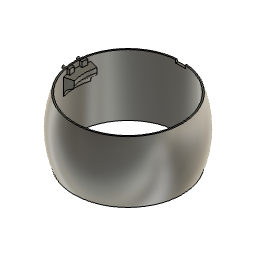
sphere_PS4_USB_C v6 (Autodesk Fusion 360 design; units mm, degrees)
Autodesk Fusion 360 part; units mm, degrees
note: some values were not read from the file. Set by a fixed rule: which face or edge a step refers to.
ref_plane "Arbeitsebene2" through (0, 0, 70) normal (0, 0, 1) x (1, 0, 0)
sketch "Skizze1" plane through (0, 0, 70) normal (0, 0, 1) x (1, 0, 0)
  circle A0 centre (0, 0) radius 60
  line L0 (-32, -65.4497) -> (-32, 74.1763) construction
  line L1 (32, -65.9786) -> (32, 70) construction
  line L2 (-70, -45) -> (87.8831, -45) construction
  line L3 (-67.6095, 45) -> (98.1964, 45) construction
  line L4 (-42.2555, 59.4219) -> (47.2161, -66.3977) construction
  line L5 (-55.8567, -78.5485) -> (54.1174, 76.1026) construction
  line L6 (5.5, 47.5) -> (-5.5, 47.5)
  line L7 (-5.5, 47.5) -> (-5.5, 72.5)
  line L8 (-5.5, 72.5) -> (5.5, 72.5)
  line L9 (5.5, 72.5) -> (5.5, 47.5)
  line L10 (5.5, 47.5) -> (-5.5, 72.5) construction
  line L11 (-5.5, 47.5) -> (5.5, 72.5) construction
  line L12 (0, 80.8433) -> (0, -85.8515) construction
  line L13 (-51.619, 47.0895) -> (-51.619, -61.7465) construction
  line L14 (19.5945, 2.5376) -> (-101.1039, -13.0936) construction
  line L15 (-57.2614, 36.8831) -> (-44.5673, -61.1352) construction
  line L16 (-101.3678, 13.1278) -> (63.9, -8.2755) construction
  line L17 (-45.9186, 50.7013) -> (-58.0992, -43.3523) construction
  point P0 (-32, 45)
  point P1 (32, -45)
  point P2 (-32, -45)
  point P3 (34.8015, 48.8759)
  point P4 (32, 45)
  point P5 (0, 60)
  point P6 (-51.619, -6.685)
  point P7 (-51.619, 6.685)
  dimension "d1" = 120
  dimension "d8" = 45
  dimension "d9" = 45
  dimension "d10" = 32
  dimension "d11" = 32
  dimension "d24" = 11
  dimension "d25" = 25
  dimension "d38" = 51.619
  dimension "d39" = 6.685
  dimension "d69" = 6.685
  constraint coincident A0.centre origin
  constraint vertical L0
  constraint vertical L1
  constraint horizontal L2
  constraint perpendicular L1 L3
  constraint coincident A0.centre L4
  constraint coincident L0 P0
  constraint coincident L3 P0
  constraint coincident L2 P1
  constraint coincident L1 P1
  constraint coincident L0 P2
  constraint coincident L2 P2
  constraint coincident L4 P0
  constraint coincident A0.centre L5
  constraint coincident A0 P3
  constraint coincident L1 P4
  constraint coincident L3 P4
  constraint coincident L5 P4
  constraint horizontal L6
  constraint perpendicular L6 L7
  constraint parallel L6 L8
  constraint parallel L7 L9
  constraint coincident L10 P5
  constraint coincident L11 P5
  constraint vertical L12
  constraint coincident A0.centre L12
  constraint coincident P5 L12
  constraint coincident A0 P5
  constraint vertical L13
  constraint coincident L13 P6
  constraint coincident P6 L14
  constraint coincident A0.centre L14
  constraint perpendicular L14 L15
  constraint coincident P6 L15
  constraint coincident A0.centre L16
  constraint coincident L16 P7
  constraint coincident L13 P7
  constraint perpendicular L16 L17
  constraint coincident P7 L17
  measures "d1" diameter of A0
  measures "d8" distance of A0.centre L3
  measures "d9" distance of A0.centre L2
  measures "d10" distance of A0.centre L1
  measures "d11" distance of A0.centre L0
  measures "d24" distance of L7 L9
  measures "d25" distance of L6 L8
  measures "d38" distance of A0.centre L13
  measures "d39" vertical distance of A0.centre P6
  measures "d69" vertical distance of A0.centre P7
sketch "Skizze4" plane through (0, 0, 0) normal (0, 1, 0) x (1, 0, 0)
  line L0 (-48.1569, -35) -> (99.3062, -35) construction
  line L1 (60.1, -70) -> (60.1, 0)
  line L2 (60.1, 0) -> (61.6, 0)
  arc A0 (61.6, -70) -> (61.6, 0) centre (-32.075, -35) ccw
  line L3 (60.1, -70) -> (61.6, -70)
  line L4 (56.0379, -68.4) -> (71.6155, -68.4) construction
  line L5 (56, -65.1) -> (73.2062, -65.1) construction
  point P0 (-32.075, -35)
  point P1 (60.1, -65.1)
  point P2 (63.2874, -65.1)
  dimension "d31" = 35
  dimension "d32" = 60.1
  dimension "d33" = 1.5
  dimension "d34" = 35
  dimension "d35" = 1.5
  dimension "d36" = 100
  dimension "d57" = 1.6
  dimension "d58" = 3.3
  dimension "d59" = 3.1874
  constraint horizontal L0
  constraint perpendicular L0 L1
  constraint horizontal L2
  constraint coincident origin L2
  constraint coincident L1.end L2.start
  constraint coincident L0 P0
  constraint coincident P0 A0.centre
  constraint horizontal L3
  constraint coincident L1.start L3.start
  constraint coincident A0.start L3.end
  constraint horizontal L4
  constraint horizontal L5
  constraint coincident L1 P1
  constraint coincident L5 P1
  constraint coincident L5 P2
  constraint coincident A0 P2
  measures "d31" distance of origin L0
  measures "d32" distance of origin L1
  measures "d33" distance of L1.end L2.end
  measures "d34" distance of L0 L3
  measures "d35" distance of L1.start A0.start
  measures "d36" radius of A0
  measures "d57" distance of A0.start L4
  measures "d58" distance of L4 L5
  measures "d59" distance of P1 P2
revolve "Drehen2" add sketch "Skizze4" angle 360 about axis through (0, 0, 1.75) along (0, 0, 1) makes body 1
ref_plane "Arbeitsebene3" through (-51.619, -6.685, 70) normal (0.991718, 0.128434, 0) x (-0.128434, 0.991718, 0)
sketch "Skizze5" plane through (-51.619, -6.685, 0) normal (0.991718, 0.128434, 0) x (-0.128434, 0.991718, 0)
  line L0 (22.1819, 67.1) -> (-34.0583, 67.1) construction
  line L1 (45.7665, 70) -> (-50, 70) construction
  line L2 (60, 70) -> (-60, 70)
  line L3 (0, -62.5) -> (0, 202.5)
  line L4 (7, 70) -> (-29, 70)
  line L5 (0, 74.3723) -> (0, 56) construction
  circle A0 centre (0, 67.1) radius 1.7
  point P0 (0, 70)
  point P1 (0, 70)
  point P2 (0, 67.1)
  dimension "d40" = 70
  dimension "d41" = 2.9
  dimension "d70" = 3.4
  constraint horizontal L0
  constraint horizontal L1
  constraint horizontal L4
  constraint coincident L1 P1
  constraint coincident L3 P1
  constraint coincident L4 P1
  constraint perpendicular L4 L5
  constraint coincident P1 L5
  constraint coincident L3 P2
  constraint coincident L0 P2
  constraint coincident P2 A0.centre
  measures "d40" distance of origin L1
  measures "d41" distance of L0 L2
  measures "d70" diameter of A0
extrude "Extrusion6" cut sketch "Skizze5" against normal blind 20 bodies 1
ref_plane "Arbeitsebene4" through (-51.619, 6.685, 70) normal (0.991718, -0.128434, 0) x (0.128434, 0.991718, 0)
sketch "Skizze8" plane through (-51.619, 6.685, 0) normal (0.991718, -0.128434, 0) x (0.128434, 0.991718, 0)
  line L0 (14, 67.1) -> (-23, 67.1) construction
  line L1 (0, 87.9567) -> (0, -11) construction
  circle A0 centre (0, 67.1) radius 1.7
  point P0 (0, 67.1)
  point P1 (0, 70)
  dimension "d74" = 3.4
  dimension "d77" = 2.9
  constraint horizontal L0
  constraint vertical L1
  constraint coincident origin L1
  constraint coincident L0 P0
  constraint coincident L1 P0
  constraint coincident P0 A0.centre
  measures "d74" diameter of A0
  measures "d77" distance of L0 P1
extrude "Extrusion7" cut sketch "Skizze8" against normal blind 20 bodies 1
extrude "Extrusion2" cut sketch "Skizze1" against normal blind 3.5 contours A0 L6 L7 L9 | A0 L7 L8 L9 picked at (-0.6119, 51.6573) bodies 1
sketch "Skizze7" plane through (0, 0, 70) normal (0, 0, 1) x (1, 0, 0)
  line L0 (48.2941, 0) -> (-42.2573, 0) construction
  line L1 (0, -37.5882) -> (0, 19.3886) construction
  circle A0 centre (0, 0) radius 60
  line L2 (5.2, 56) -> (-5.2, 56)
  line L3 (-5.2, 56) -> (-5.2, 64)
  line L4 (-5.2, 64) -> (5.2, 64)
  line L5 (5.2, 64) -> (5.2, 56)
  line L6 (78.9842, -6.685) -> (-85, -6.685) construction
  line L7 (-51.619, -63.2499) -> (-51.619, 65) construction
  line L8 (78.5823, 6.685) -> (-93.603, 6.685) construction
  line L9 (25.1933, 3.2627) -> (-82.471, -10.6805) construction
  line L10 (13.8036, -1.7877) -> (-78.099, 10.1143) construction
  line L11 (-48.2585, -9.2749) -> (-54.2089, -10.0455)
  line L12 (-54.2089, -10.0455) -> (-54.9795, -4.0951)
  line L13 (-54.9795, -4.0951) -> (-49.0291, -3.3245)
  line L14 (-49.0291, -3.3245) -> (-48.2585, -9.2749)
  line L15 (-48.2585, 9.2749) -> (-54.2089, 10.0455)
  line L16 (-54.2089, 10.0455) -> (-54.9795, 4.0951)
  line L17 (-54.9795, 4.0951) -> (-49.0291, 3.3245)
  line L18 (-49.0291, 3.3245) -> (-48.2585, 9.2749)
  line L19 (-54.363, -8.8554) -> (-56.3464, -9.1123)
  line L20 (-56.3464, -9.1123) -> (-56.8088, -5.5421)
  line L21 (-56.8088, -5.5421) -> (-54.8253, -5.2852)
  line L22 (-54.8253, -5.2852) -> (-54.363, -8.8554)
  line L23 (-54.8253, 5.2852) -> (-56.8088, 5.5421)
  line L24 (-56.8088, 5.5421) -> (-56.3464, 9.1123)
  line L25 (-56.3464, 9.1123) -> (-54.363, 8.8554)
  line L26 (-54.363, 8.8554) -> (-54.8253, 5.2852)
  line L27 (15.5391, 4.1637) -> (-82.6757, -22.1529) construction
  line L28 (7.2575, -1.9447) -> (-68.8486, 18.4479) construction
  line L29 (-48.2963, 12.941) -> (-57.9555, 15.5291)
  arc A1 (-48.2963, 12.941) -> (-48.2963, -12.941) centre (0, 0) ccw
  line L30 (-48.2963, -12.941) -> (-57.9555, -15.5291)
  line L31 (-56.1923, 10.3023) -> (-59.0434, 10.6716)
  line L32 (-56.9629, 4.352) -> (-56.1923, 10.3023)
  line L33 (-56.9629, 4.352) -> (-59.814, 4.7212)
  line L34 (-56.1923, -10.3023) -> (-59.0434, -10.6716)
  line L35 (-56.9629, -4.352) -> (-59.814, -4.7212)
  line L36 (-56.1923, -10.3023) -> (-56.9629, -4.352)
  point P0 (-51.619, -6.685)
  point P1 (-51.619, 6.685)
  point P2 (-57.9555, -15.5291)
  point P3 (-57.9555, 15.5291)
  dimension "d60" = 120
  dimension "d61" = 5.2
  dimension "d62" = 5.2
  dimension "d63" = 64
  dimension "d64" = 8
  dimension "d78" = 6.685
  dimension "d79" = 51.619
  dimension "d80" = 6.685
  dimension "d81" = 3
  dimension "d82" = 3
  dimension "d83" = 3
  dimension "d84" = 3
  dimension "d85" = 3
  dimension "d86" = 3
  dimension "d87" = 3
  dimension "d88" = 3
  dimension "d89" = 1.8
  dimension "d90" = 1.8
  dimension "d91" = 2
  dimension "d92" = 1.8
  dimension "d93" = 1.8
  dimension "d94" = 2
  dimension "d95" = 15
  dimension "d96" = 15
  dimension "d97" = 10
  constraint horizontal L0
  constraint coincident A0.centre L0
  constraint vertical L1
  constraint coincident A0.centre L1
  constraint coincident A0.centre A1.centre
  constraint horizontal L2
  constraint vertical L3
  constraint horizontal L4
  constraint vertical L5
  constraint horizontal L6
  constraint vertical L7
  constraint horizontal L8
  constraint coincident L6 P0
  constraint coincident L7 P0
  constraint coincident L8 P1
  constraint coincident L7 P1
  constraint coincident P1 L10
  constraint coincident A0.centre L10
  constraint coincident A0.centre L9
  constraint coincident P0 L9
  constraint perpendicular L11 L12
  constraint parallel L11 L13
  constraint parallel L12 L14
  constraint parallel L9 L11
  constraint perpendicular L15 L16
  constraint parallel L15 L17
  constraint parallel L16 L18
  constraint parallel L10 L17
  constraint perpendicular L19 L20
  constraint parallel L19 L21
  constraint parallel L20 L22
  constraint parallel L12 L22
  constraint perpendicular L23 L24
  constraint parallel L23 L25
  constraint parallel L24 L26
  constraint parallel L16 L26
  constraint coincident L16 L25.end
  constraint coincident L12 L21.end
  constraint coincident A0.centre L27
  constraint coincident A0.centre L28
  constraint coincident L27 P2
  constraint coincident A0 P2
  constraint coincident A0 P3
  constraint coincident L28 P3
  constraint coincident P3 L29.end
  constraint coincident L28 L29.start
  constraint coincident P2 L30.end
  constraint parallel L27 L30
  constraint coincident L15 L31.start
  constraint parallel L15 L31
  constraint parallel L24 L32
  constraint coincident L23.end L32
  constraint coincident L31.start L32
  constraint coincident L31 L32.end
  constraint parallel L17 L33
  constraint coincident L17 L32.start
  constraint coincident L32 L33.start
  constraint coincident L32.start L33
  constraint coincident A0 L31.end
  constraint coincident A0 L33.end
  constraint parallel L13 L35
  constraint parallel L11 L34
  constraint coincident L11 L34.start
  constraint coincident L13 L35.start
  constraint parallel L20 L36
  constraint coincident L19.end L36
  constraint coincident L35.start L36
  constraint coincident L34.start L36
  constraint coincident L34 L36.start
  constraint coincident L35 L36.end
  constraint coincident A0 L35.end
  constraint coincident A0 L34.end
  measures "d60" diameter of A0
  measures "d61" distance of L1 L2.start
  measures "d62" distance of L1 L3
  measures "d63" distance of A0.centre L4
  measures "d64" distance of L2 L4
  measures "d78" distance of A0.centre L6
  measures "d79" distance of A0.centre L7
  measures "d80" distance of A0.centre L8
  measures "d81" distance of P0 L12
  measures "d82" distance of P0 L14
  measures "d83" distance of P0 L13
  measures "d84" distance of P0 L11
  measures "d85" distance of P1 L18
  measures "d86" distance of P1 L16
  measures "d87" distance of P1 L15
  measures "d88" distance of P1 L17
  measures "d89" distance of P0 L21
  measures "d90" distance of P0 L19
  measures "d91" distance of L20 L22
  measures "d92" distance of P1 L23
  measures "d93" distance of P1 L25
  measures "d94" distance of L24 L26
  measures "d95" angle of L0 L27
  measures "d96" angle of L0 L28
  measures "d97" distance of P3 L29.start
extrude "Extrusion4" add sketch "Skizze7" along normal blind 1.6 separate body makes body 2
extrude "Extrusion5" add sketch "Skizze7" against normal blind 3.5 contours A0 L3 L4 L5 | A0 L2 L3 L5 bodies 2
extrude "Extrusion8" add sketch "Skizze7" against normal blind 6 contours L15 L16 L17 L26 A1 | L15 L17 L18 A1 | L11 L12 L13 L22 A1 | L11 L13 L14 A1 bodies 2
extrude "Extrusion9" add sketch "Skizze7" against normal blind 4.8 contours L16 L23 L24 L25 L26 L32 | L12 L19 L20 L21 L22 L36 bodies 2
extrude "Extrusion10" cut sketch "Skizze7" against normal blind 1.2 contours L16 L23 L24 L25 L26 L32 | L12 L19 L20 L21 L22 L36 bodies 2
extrude "Extrusion11" add sketch "Skizze7" against normal blind 6 separate body contours A0 L24 L31 L32 L33 | A0 L20 L34 L35 L36 makes body 3 at (-59.545, 7.3752, 66) makes body 4 at (-59.4593, -8.0366, 66)
extrude "Extrusion12" cut sketch "Skizze7" against normal blind 0.2 contours A0 L24 L31 L32 L33 | A0 L20 L34 L35 L36 bodies 3 4
extrude "Extrusion13" add sketch "Skizze5" against normal blind 14.5 bodies 4
extrude "Extrusion14" cut sketch "Skizze5" against normal blind 5 bodies 4
fillet "Abrundung1" radius 0.5 1 edges at (-65.7953, -10.1191, 67.7147) on bodies 4
move_face "Flächen versetzen1" offset -0.15 1 faces at (-61.5514, -7.585, 68.7563) on bodies 4
extrude "Extrusion15" add sketch "Skizze8" against normal blind 14.5 bodies 3
extrude "Extrusion16" cut sketch "Skizze8" against normal blind 5 bodies 3
fillet "Abrundung2" radius 0.5 1 edges at (-66.2025, 6.9755, 67.7147) on bodies 3
move_face "Flächen versetzen2" offset -0.15 1 faces at (-63.2774, 9.9045, 66.9758) on bodies 3
extrude "Extrusion17" add sketch "Skizze7" against normal blind 16 separate body contours A0 L15 L16 L25 L29 A1 L31 L32 | A0 L24 L31 L32 L33 | A0 L12 L13 L16 L17 L21 L23 A1 L32 L33 L35 L36 | L15 L16 L17 L26 A1 | A0 L20 L34 L35 L36 | L16 L23 L24 L25 L26 L32 | A0 L11 L12 L19 A1 L30 L34 L36 | L11 L12 L13 L22 A1 | L12 L19 L20 L21 L22 L36 makes body 5
move_face "Flächen versetzen4" offset -6 1 faces at (-56.5584, -3.2438, 70) on bodies 5
move_face "Flächen versetzen3" offset 0.1 5 faces at (-58.6097, 12.8416, 57.3333) (-59.1583, 10.0146, 60.6667) (-59.9426, -2.6248, 57.3333) (-59.4593, -8.0366, 57.3333) (-58.9424, -11.2155, 60.6667) on bodies 5
combine "Kombinieren1" operation add target body 1 tool bodies 5
fillet "Abrundung3" radius 5 1 edges at (-50, 0, 54) on bodies 1
fillet "Abrundung4" radius 10 1 edges at (-60.1, 0, 54) on bodies 1
hidden bodies 2
named bodies: "housing", "pcb", "knob1", "knob2"
